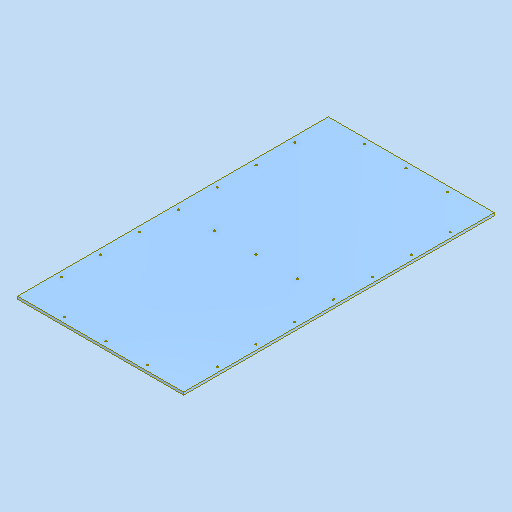
# Autodesk Inventor part: нижняя плита
Saved by Autodesk Inventor 2025 (Build 290162000, 162)
## iProperties
Created: 2025-01-21
Part Number: нижняя плита
Material: Алюминий 6061
Document SubType Name: Modeling
Designer: volko
Density: 2.7 g/cm^3
Appearance: Алюминий — плоский
Mass: 2416.26 g
Surface Area: 3692.3 cm^2
Volume: 894.911 cm^3
Author: volko
Autodesk Inventor part; units mm, degrees
ref_plane "YZ Plane" through (0, 0, 0) normal (1, 0, 0) x (0, 1, 0)
ref_plane "XZ Plane" through (0, 0, 0) normal (0, 1, 0) x (-1, 0, 0)
ref_plane "XY Plane" through (0, 0, 0) normal (0, 0, 1) x (1, 0, 0)
sketch "Эскиз1" plane through (0, 0, 0) normal (0, 1, 0) x (-1, 0, 0)
  line L0 (0, 290) -> (155, 290)
  line L1 (155, 290) -> (155, -290)
  line L2 (0, 290) -> (0, 0)
  line L3 (0, 0) -> (200, 0)
  line L4 (0, 290) -> (-155, 290)
  line L5 (-155, 290) -> (-155, -290)
  line L6 (0, -290) -> (155, -290)
  line L7 (155, -290) -> (155, -125)
  line L8 (-155, -290) -> (-155, -125)
  line L9 (0, -290) -> (-155, -290)
  point P0 (155, 125)
  point P1 (-155, 125)
  dimension "d3" = 310
  dimension "d6" = 580
  constraints: 20 end point, 7 symmetric about line, 4 point on line, 1 vertical
  measures "d3" distance between parallel lines of L5 L1
  measures "d6" distance between parallel lines of L4 L9
extrude "Выдавливание1" add sketch "Эскиз1" along normal blind 5
sketch "Эскиз2" plane through (0, 0, 0) normal (0, 1, 0) x (1, 0, 0)
  line L0 (-155, -290) -> (155, -290) projected
  line L1 (155, -290) -> (155, 290) projected
  point P0 (0, 0)
  point P1 (77.5, -280)
  point P2 (0, -280)
  point P3 (-77.5, -280)
  point P4 (77.5, 0)
  point P5 (0, 0)
  point P6 (-77.5, 0)
  point P7 (77.5, 280)
  point P8 (0, 280)
  point P9 (-77.5, 280)
  point P10 (145, -217.5)
  point P11 (145, -145)
  point P12 (145, -72.5)
  point P13 (145, 0)
  point P14 (145, 72.5)
  point P15 (145, 145)
  point P16 (145, 217.5)
  point P17 (-145, -217.5)
  point P18 (-145, -145)
  point P19 (-145, -72.5)
  point P20 (-145, 0)
  point P21 (-145, 72.5)
  point P22 (-145, 145)
  point P23 (-145, 217.5)
  dimension "d15" = 10
  dimension "d16" = 77.5
  dimension "d19" = 77.5
  dimension "d22" = 280
  dimension "d25" = 10
  dimension "d26" = 72.5
  dimension "d29" = 72.5
  dimension "d32" = 290
  constraints: 2 horizontal, 2 vertical, 21 other
  measures "d15" distance from line of L0 point (77.5, -280)
  measures "d16" distance from line of point (77.5, -280) L1
  measures "d19" distance of point (77.5, -280) point (0, -280)
  measures "d22" distance of point (77.5, -280) point (77.5, 0)
  measures "d25" distance from line of point (145, -217.5) L1
  measures "d26" distance from line of L0 point (145, -217.5)
  measures "d29" distance of point (145, -217.5) point (145, -145)
  measures "d32" distance of point (145, -217.5) point (-145, -217.5)
hole "Отверстие2" at (77.5, 0, 280) at (0, 0, 280) at (-77.5, 0, 280) at (77.5, 0, 0) at (0, 0, 0) at (-77.5, 0, 0) at (77.5, 0, -280) at (0, 0, -280) at (-77.5, 0, -280) at (145, 0, 217.5) at (145, 0, 145) at (145, 0, 72.5) at (145, 0, 0) at (145, 0, -72.5) at (145, 0, -145) at (145, 0, -217.5) at (-145, 0, 217.5) at (-145, 0, 145) at (-145, 0, 72.5) at (-145, 0, 0) at (-145, 0, -72.5) at (-145, 0, -145) at (-145, 0, -217.5) direction (0, 1, 0) diameter 3 end through all countersink diameter 11 countersink angle 90
